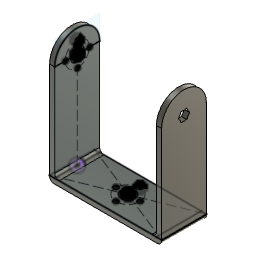
servo U stand v2 v3 (Autodesk Fusion 360 design; units mm, degrees)
Autodesk Fusion 360 part; units mm, degrees
note: some values were not read from the file. Set by a fixed rule: which sketch regions a step uses.
sketch "Sketch1" plane through (0, 0, 0) normal (0, 0, 1) x (1, 0, 0)
  line L0 (32.5, -13) -> (-32.5, -13)
  line L1 (-32.5, -13) -> (-32.5, 13)
  line L2 (-32.5, 13) -> (32.5, 13)
  line L3 (32.5, 13) -> (32.5, -13)
  line L4 (32.5, -13) -> (-32.5, 13) construction
  line L5 (-32.5, -13) -> (32.5, 13) construction
  line L6 (-29.5, -13) -> (-29.5, 13)
  line L7 (29.5, 13) -> (29.5, -13)
  circle A0 centre (0, 0) radius 4
  circle A1 centre (0, 0) radius 7 construction
  circle A2 centre (0, 7) radius 1.25
  line L8 (0, 0) -> (0, 7) construction
  circle A3 centre (-7, 0) radius 1.25
  circle A4 centre (0, -7) radius 1.25
  circle A5 centre (7, 0) radius 1.25
  dimension "d3" = 65
  dimension "d5" = 26
  dimension "d6" = 3
  dimension "d7" = 3
  dimension "d8" = 8
  dimension "d9" = 14
  dimension "d10" = 2.5
  dimension "d12" = 360
  constraint horizontal L0
  constraint perpendicular L0 L1
  constraint parallel L0 L2
  constraint parallel L1 L3
  constraint coincident L4 A0.centre
  constraint coincident L5 A0.centre
  constraint coincident A0.centre A1.centre
  constraint coincident L0 L6.start
  constraint coincident L2 L6.end
  constraint perpendicular L2 L6
  constraint coincident L2 L7.start
  constraint coincident L0 L7.end
  constraint perpendicular L0 L7
  constraint coincident A1 A2.centre
  constraint vertical L8
  constraint coincident A2.centre L8.end
  measures "d3" distance of L0.start L0.end
  measures "d5" distance of L0.end L1.end
  measures "d6" distance of L1 L6
  measures "d7" distance of L3 L7
  measures "d8" diameter of A0
  measures "d9" diameter of A1
  measures "d10" diameter of A2
extrude "Extrude1" add sketch "Sketch1" against normal blind 3
extrude "Extrude2" add sketch "Sketch1" along normal blind 70 contours L0 L2 L3 L7 | L0 L1 L2 L6
sketch "Sketch2" plane through (-29.5, 0, 0) normal (1, 0, 0) x (0, 1, 0)
  line L0 (-13, 0) -> (13, 0)
  line L1 (13, 0) -> (13, 70)
  line L2 (13, 70) -> (-13, 70)
  line L3 (-13, 70) -> (-13, 0)
  line L4 (0, 0) -> (0, 56) construction
  circle A0 centre (0, 56) radius 7 construction
  circle A1 centre (0, 56) radius 4
  circle A2 centre (0, 63) radius 1.25
  line L5 (0, 56) -> (0, 63) construction
  circle A3 centre (-7, 56) radius 1.25
  circle A4 centre (0, 49) radius 1.25
  circle A5 centre (7, 56) radius 1.25
  line L6 (0, 56) -> (13, 56)
  line L7 (0, 56) -> (-13, 56)
  arc A6 (13, 56) -> (-13, 56) centre (0, 56) ccw
  line L8 (1.5877, 58.75) -> (-1.5877, 58.75)
  line L9 (-1.5877, 58.75) -> (-3.1754, 56)
  line L10 (-3.1754, 56) -> (-1.5877, 53.25)
  line L11 (-1.5877, 53.25) -> (1.5877, 53.25)
  line L12 (1.5877, 53.25) -> (3.1754, 56)
  line L13 (3.1754, 56) -> (1.5877, 58.75)
  point P0 (0, 56)
  dimension "d18" = 56
  dimension "d19" = 14
  dimension "d20" = 8
  dimension "d21" = 2.5
  dimension "d23" = 360
  dimension "d24" = 26
  dimension "d29" = 2.75
  constraint coincident L4.start origin
  constraint perpendicular L2 L4
  constraint coincident P0 L4.end
  constraint concentric A0 A1
  constraint coincident A0 A2.centre
  constraint parallel L4 L5
  constraint coincident A2.centre L5.end
  constraint concentric A0 A6
  constraint perpendicular L1 L6
  constraint perpendicular L3 L7
  constraint horizontal L8
  measures "d18" distance of L4.start P0
  measures "d19" diameter of A0
  measures "d20" diameter of A1
  measures "d21" diameter of A2
  measures "d24" diameter of A6
  measures "d29" distance of P0 L13
extrude "Extrude3" cut sketch "Sketch2" against normal through all contours L1 L2 L3 A6 | A3 L7 | A3 L7 | A5 L6 | A5 L6 | A1 L6 L7 L10 L11 L12 | A1 L6 L7 L8 L9 L13 | L6 L7 L8 L9 L13 | L6 L7 L10 L11 L12 | A2 | A4
fillet "Fillet1" radius 2.5 4 edges at (32.5, 0, -3) (29.5, 0, 0) (-29.5, 0, 0) (-32.5, 0, -3)
extrude "Extrude4" cut sketch "Sketch2" along normal blind 67 contours L1 L2 L3 A6 | L6 L7 L8 L9 L13 | L6 L7 L10 L11 L12
equation "width = 26 mm"
equation "thickness = 3 mm"
equation "d3 = length"
equation "length = 65 mm"
equation "d5 = width"
equation "d6 = thickness"
equation "d7 = thickness"
equation "d13 = -thickness"
equation "height = 70 mm"
equation "d16 = height"
equation "d18 = height - 14 mm"
